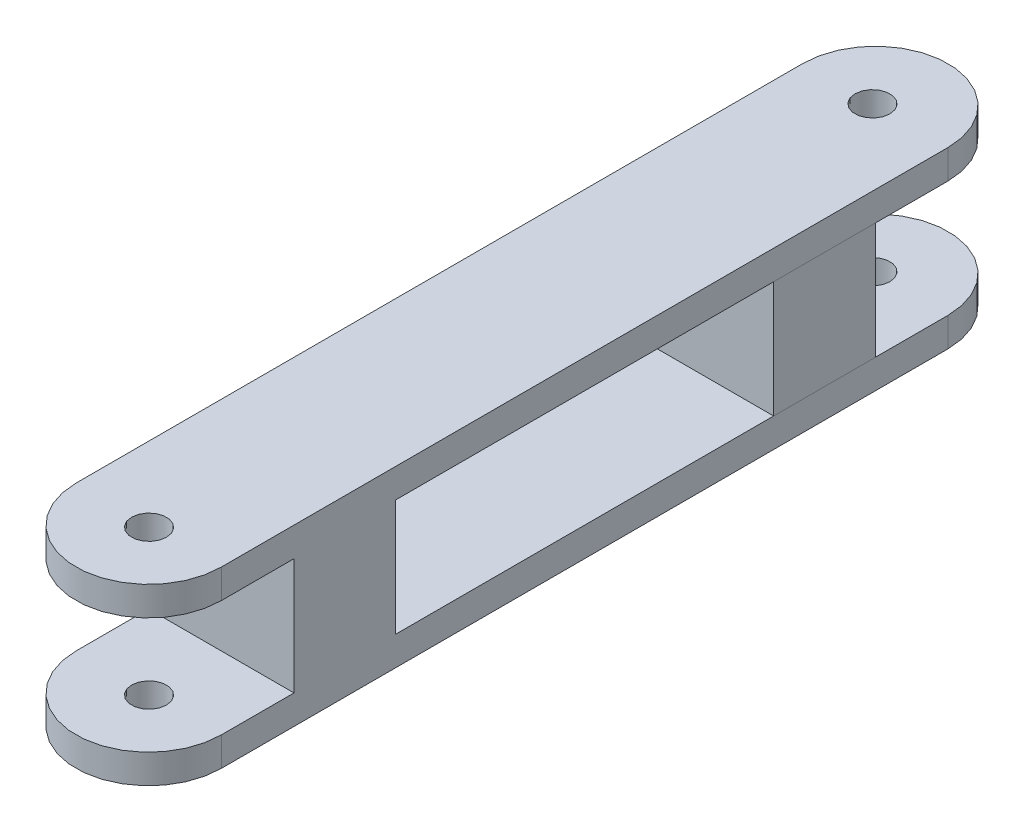
AgriRover_Armupperlink (Autodesk Fusion 360 design; units mm, degrees)
part number: 2026-09-20-15-53-34-513
Autodesk Fusion 360 part; units mm, degrees
sketch "Sketch1" plane through (0, 0, 0) normal (0, 0, 1) x (1, 0, 0)
  line L0 (-50, 50) -> (-25, 50)
  line L1 (-25, 50) -> (-25, -75)
  line L2 (-25, -75) -> (-50, -75)
  line L3 (-50, -75) -> (-50, 50)
  circle A0 centre (-37.5, -75) radius 12.5
  circle A1 centre (-37.5, 50) radius 12.5
  constraint horizontal L0
  constraint vertical L1
  constraint horizontal L2
  constraint vertical L3
  constraint midpoint L2 A0.centre
  constraint coincident L1.end A0
  constraint midpoint L0 A1.centre
  constraint coincident L0.end A1
extrude "Extrude1" add sketch "Sketch1" along normal blind 30
sketch "Sketch2" plane through (-25, 0, 0) normal (1, 0, 0) x (0, 1, 0)
  line L0 (-75, 0) -> (50, 0)
  line L1 (50, 0) -> (50, 30)
  line L2 (50, 30) -> (-75, 30)
  line L3 (-75, 30) -> (-75, 0)
  line L4 (-75, 25) -> (-45, 25)
  line L5 (-45, 25) -> (-45, 5)
  line L6 (-45, 5) -> (-75, 5)
  line L7 (-75, 5) -> (-75, 25)
  line L8 (-35, 25) -> (10, 25)
  line L9 (10, 25) -> (10, 5)
  line L10 (10, 5) -> (-35, 5)
  line L11 (-35, 5) -> (-35, 25)
  line L12 (20, 25) -> (50, 25)
  line L13 (50, 25) -> (50, 5)
  line L14 (50, 5) -> (20, 5)
  line L15 (20, 5) -> (20, 25)
  constraint horizontal L4
  constraint vertical L5
  constraint horizontal L6
  constraint vertical L7
  constraint coincident L3 L4.start
  constraint horizontal L8
  constraint vertical L9
  constraint horizontal L10
  constraint vertical L11
  constraint horizontal L12
  constraint vertical L13
  constraint horizontal L14
  constraint vertical L15
  constraint coincident L1 L13.end
extrude "Extrude2" cut sketch "Sketch2" against normal blind 100 contours L3 L4 L5 L6 L7 | L1 L12 L13 L14 L15 | L8 L9 L10 L11
extrude "Extrude3" add 1 faces at (-33.3333, -35, 11.6667) along direction (0, 1, 0) blind 5
extrude "Extrude4" add 1 faces at (-33.3333, 10, 18.3333) along direction (0, -1, 0) blind 5
extrude "Extrude5" add 1 faces at (-33.3333, 50, 11.6667) along direction (0, -1, 0) blind 5
extrude "Extrude6" add 1 faces at (-33.3333, -75, 18.3333) along direction (0, 1, 0) blind 5
sketch "Sketch3" plane through (0, 45, 0) normal (0, -1, 0) x (1, 0, 0)
  line L0 (-50, 25) -> (-50, 5)
  line L1 (-50, 5) -> (-25, 5)
  line L2 (-25, 5) -> (-25, 25)
  line L3 (-25, 25) -> (-50, 25)
  line L4 (-50, 23) -> (-25, 23)
  line L5 (-25, 23) -> (-25, 6)
  line L6 (-25, 6) -> (-50, 6)
  line L7 (-50, 6) -> (-50, 23)
  constraint horizontal L4
  constraint vertical L5
  constraint horizontal L6
  constraint vertical L7
  constraint coincident L2 L5.end
  constraint coincident L0 L4.start
extrude "Extrude7" cut sketch "Sketch3" against normal blind 100 contours L0 L2 L4 L5 L6 L7
extrude "Extrude8" cut 1 faces at (-41.6667, 46.6667, 23) along direction (0, 0, 1) blind 2
extrude "Extrude9" cut 1 faces at (-38.4272, 54.0622, 6) along direction (0, 0, -1) blind 1
sketch "Sketch4" plane through (0, 0, 30) normal (0, 0, 1) x (-1, 0, 0)
  arc A0 (50, 75) -> (25, 75) centre (37.5, 75) ccw
  line L0 (25, 75) -> (25, -50)
  arc A1 (25, -50) -> (50, -50) centre (37.5, -50) ccw
  line L1 (50, -50) -> (50, 75)
sketch "Sketch5" plane through (0, -70, 0) normal (0, 1, 0) x (-1, 0, 0)
  line L0 (50, 5) -> (50, 25)
  line L1 (50, 25) -> (25, 25)
  line L2 (25, 25) -> (25, 5)
  line L3 (25, 5) -> (50, 5)
  line L4 (25, 23) -> (50, 23)
  line L5 (50, 23) -> (50, 6)
  line L6 (50, 6) -> (25, 6)
  line L7 (25, 6) -> (25, 23)
  constraint horizontal L4
  constraint vertical L5
  constraint horizontal L6
  constraint vertical L7
  constraint coincident L0 L5.end
  constraint coincident L2 L4.start
extrude "Extrude10" cut sketch "Sketch5" against normal blind 100 contours L0 L2 L4 L5 L6 L7
extrude "Extrude11" cut 1 faces at (-41.6667, -71.6667, 6) along direction (0, 0, -1) blind 1
extrude "Extrude12" cut 1 faces at (-38.5657, -80.9114, 23) along direction (0, 0, 1) blind 2
sketch "Sketch6" plane through (0, 0, 30) normal (0, 0, 1) x (-1, 0, 0)
  circle A0 centre (37.1481, 75.2839) radius 3
  circle A1 centre (38, -50) radius 3
  dimension "d25" = 6
  measures "d25" diameter of A0
extrude "Extrude13" cut sketch "Sketch6" against normal blind 100
sketch "Sketch7" plane through (0, 0, 25) normal (0, 0, -1) x (1, 0, 0)
  circle A0 centre (-38, -50) radius 3
  line L0 (-25, -50) -> (-25, -20)
  line L1 (-25, -20) -> (-50, -20)
  line L2 (-50, -20) -> (-50, -50)
  arc A1 (-50, -50) -> (-25, -50) centre (-37.5, -50) ccw
  circle A2 centre (-37.5, -50) radius 12.5
  line L3 (-50, -37.5) -> (-25, -37.5)
  constraint concentric A1 A2
  constraint tangent L0 A2
  constraint coincident L2 L3.start
  constraint coincident L0 L3.end
  constraint perpendicular L0 L3
  constraint tangent A2 L3
extrude "Extrude14" cut 1 faces at (-33.3333, 20, 11.6667) along direction (0, -1, 0) blind 20
extrude "Extrude15" add sketch "Sketch7" along normal blind 20 contours L0 L1 L2 L3
sketch "Sketch8" plane through (0, 0, 0) normal (0, 0, -1) x (1, 0, 0)
  circle A0 centre (-38, -50) radius 3
  circle A1 centre (-37.1481, 75.2839) radius 3
  arc A2 (-25, 75) -> (-50, 75) centre (-37.5, 75) ccw
  line L0 (-50, 75) -> (-50, -50)
  arc A3 (-50, -50) -> (-25, -50) centre (-37.5, -50) ccw
  line L1 (-25, -50) -> (-25, 75)
sketch "Sketch9" plane through (0, 0, 25) normal (0, 0, -1) x (1, 0, 0)
  circle A0 centre (-37.1481, 75.2839) radius 3
  line L0 (-50, 75) -> (-50, 45)
  line L1 (-50, 45) -> (-25, 45)
  line L2 (-25, 45) -> (-25, 75)
  arc A1 (-25, 75) -> (-50, 75) centre (-37.5, 75) ccw
  circle A2 centre (-37.5, 75) radius 12.5
  line L3 (-50, 62.5) -> (-25, 62.5)
  line L4 (-50, 62.5) -> (-25, 62.5)
  line L5 (-25, 62.5) -> (-25, 45)
  line L6 (-25, 45) -> (-50, 45)
  line L7 (-50, 45) -> (-50, 62.5)
  constraint concentric A1 A2
  constraint coincident L0 L3.start
  constraint coincident L2 L3.end
  constraint perpendicular L2 L3
  constraint tangent A2 L3
  constraint horizontal L4
  constraint vertical L5
  constraint horizontal L6
  constraint vertical L7
  constraint coincident L1.end L2.start
extrude "Extrude16" cut 1 faces at (-33.3333, -45, 18.3333) along direction (0, 1, 0) blind 20
extrude "Extrude17" add sketch "Sketch9" along normal blind 20 contours L0 L1 L2 L3 L4 L5 L6 L7
sketch "Sketch10" plane through (0, 0, 25) normal (0, 0, -1) x (1, 0, 0)
  line L0 (-25, 45) -> (-50, 45)
  line L1 (-50, 45) -> (-50, -20)
  line L2 (-50, -20) -> (-25, -20)
  line L3 (-25, -20) -> (-25, 45)
  line L4 (-50, -10) -> (-25, -10)
  line L5 (-25, -10) -> (-25, -1)
  line L6 (-25, -1) -> (-50, -1)
  line L7 (-50, -1) -> (-50, -10)
  line L8 (-50, 35) -> (-25, 35)
  line L9 (-25, 35) -> (-25, 26)
  line L10 (-25, 26) -> (-50, 26)
  line L11 (-50, 26) -> (-50, 35)
  constraint horizontal L4
  constraint vertical L5
  constraint horizontal L6
  constraint vertical L7
  constraint coincident L3 L5.end
  constraint coincident L1 L4.start
  constraint horizontal L8
  constraint vertical L9
  constraint horizontal L10
  constraint vertical L11
  constraint coincident L3 L9.end
  constraint coincident L1 L8.start
extrude "Extrude18" add sketch "Sketch10" along normal blind 20 contours L1 L3 L8 L9 L10 L11 | L1 L3 L4 L5 L6 L7
sketch "Sketch11" plane through (-50, 0, 0) normal (-1, 0, 0) x (0, -1, 0)
  line L0 (-1, 25) -> (26, 25)
  line L1 (26, 25) -> (26, 5)
  line L2 (26, 5) -> (-1, 5)
  line L3 (-1, 5) -> (-1, 25)
  line L4 (35, 25) -> (45, 25)
  line L5 (45, 25) -> (45, 5)
  line L6 (45, 5) -> (35, 5)
  line L7 (35, 5) -> (35, 25)
  line L8 (-10, 25) -> (-10, 5)
  line L9 (-10, 5) -> (-20, 5)
  line L10 (-20, 5) -> (-20, 25)
  line L11 (-20, 25) -> (-10, 25)
  line L12 (62.5, 5) -> (62.5, 25)
  line L13 (62.5, 25) -> (75, 25)
  line L14 (75, 25) -> (75, 30)
  line L15 (75, 30) -> (-50, 30)
  line L16 (-50, 30) -> (-50, 25)
  line L17 (-50, 25) -> (-37.5, 25)
  line L18 (-37.5, 25) -> (-37.5, 5)
  line L19 (-37.5, 5) -> (-50, 5)
  line L20 (-50, 5) -> (-50, 0)
  line L21 (-50, 0) -> (75, 0)
  line L22 (75, 0) -> (75, 5)
  line L23 (75, 5) -> (62.5, 5)
  line L24 (-10, 25) -> (45, 25)
  line L25 (45, 25) -> (45, 5)
  line L26 (45, 5) -> (-10, 5)
  line L27 (-10, 5) -> (-10, 25)
  constraint horizontal L24
  constraint vertical L25
  constraint horizontal L26
  constraint vertical L27
  constraint coincident L5.end L6.start
  constraint coincident L8.start L11.end
extrude "Extrude19" cut sketch "Sketch11" against normal blind 100 contours L3 L8 L24 L26 L27 | L1 L7 L24 L26
